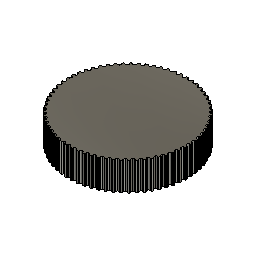
gear_67z (Autodesk Fusion 360 design; units mm, degrees)
Autodesk Fusion 360 part; units mm, degrees
sketch "Sketch1" plane through (0, 0, 0) normal (0, 0, 1) x (1, 0, 0) in component "gt2 pulley"
  circle A0 centre (0, 0) radius 21.3268 construction
  circle A1 centre (0, 0) radius 20.3228 construction
  line L0 (0, 0) -> (0, 21.3268) construction
  line L1 (0, 0) -> (0.9996, 21.3033) construction
  line L2 (0, 0) -> (1.4057, 21.2804) construction
  circle A2 centre (0, 0) radius 21.0728 construction
  arc A3 (0.3932, 20.9351) -> (0.4668, 20.6401) centre (1.389, 21.0269) ccw
  circle A4 centre (0, 0) radius 20.9228 construction
  arc A5 (0.2455, 21.0713) -> (0, 21.0728) centre (0, 0) ccw
  arc A6 (0.3932, 20.9351) -> (0.2455, 21.0713) centre (0.2438, 20.9213) ccw
  arc A7 (0.4668, 20.6401) -> (0.9526, 20.3004) centre (0.9786, 20.8548) ccw
  arc A8 (0, 21.0728) -> (-0.2455, 21.0713) centre (0, 0) ccw
  arc A9 (-0.2455, 21.0713) -> (-0.3932, 20.9351) centre (-0.2438, 20.9213) ccw
  arc A10 (-0.4668, 20.6401) -> (-0.3932, 20.9351) centre (-1.389, 21.0269) ccw
  arc A11 (-0.9524, 20.3004) -> (-0.4668, 20.6401) centre (-0.9786, 20.8548) ccw
  arc A12 (0.9526, 20.3004) -> (-0.9526, 20.3004) centre (0, 0) ccw
  point P0 (1.389, 21.0269)
  point P1 (0, 21.0728)
  dimension "d18" = 42.6535
  dimension "d19" = 2.687
  dimension "d22" = 1.004
  dimension "d24" = 0.75
  dimension "d26" = 1
  dimension "d27" = 0.15
  dimension "d28" = 0.15
  dimension "d47" = 0.555
  dimension "d52" = 3.812
  constraint coincident A0.centre A1.centre
  constraint coincident A0 L0.end
  constraint vertical L0
  constraint coincident A0 L1.end
  constraint coincident A0 L2.end
  constraint concentric A1 A2
  constraint coincident A1 A7.end
  constraint coincident L1 A7.end
  constraint coincident A2 P0
  constraint coincident L2 P0
  constraint coincident P0 A3.centre
  constraint coincident A2 P1
  constraint coincident L0 P1
  constraint concentric A2 A4
  constraint coincident P1 A5.end
  constraint coincident A4 A6.centre
  constraint coincident A3.start A6.start
  constraint tangent A3 A6
  constraint tangent A3 A7
  constraint symmetric L0 A7.end A12.end
  constraint symmetric L0 A3.start A9.end
  constraint symmetric L0 A3.end A10.start
  constraint symmetric L0 A3 A10
  constraint symmetric L0 A5.start A8.end
  constraint symmetric L0 P1 A5.end
  constraint symmetric L0 A5 A8
  constraint symmetric L0 A6 A9
  constraint symmetric L0 A7 A11
  constraint coincident A1 A11.start
  constraint tangent A1 A7
  constraint coincident L1 A7.centre
  measures "d18" diameter of A0
  measures "d19" angle of L0 L1
  measures "d22" distance of A0 A1
  measures "d24" distance of A1 A2
  measures "d26" radius of A3
  measures "d27" distance of A2 A4
  measures "d28" radius of A6
  measures "d47" radius of A7
extrude "Extrude1" add sketch "Sketch1" along normal blind 10 makes body 1
pattern_circular "C-Pattern1" count 67 over 360 about axis through (0, 0, 1.75) along (0, 0, 1) of bodies 1 makes body 2 at (-2.6393, 20.1506, 6.6667) makes body 3 at (-4.5147, 19.815, 6.6667) makes body 4 at (-6.3503, 19.3051, 6.6667) makes body 5 at (-7.5442, 18.8706, 6.6667) makes body 6 at (-9.2781, 18.0813, 6.6667) makes body 7 at (-10.2072, 17.5735, 3.3333) makes body 8 at (-12.9818, 15.6361, 6.6667) makes body 9 at (-14.3889, 14.3518, 6.6667) makes body 10 at (-15.2575, 13.4247, 6.6667) makes body 11 at (-16.8126, 11.4171, 6.6667) makes body 12 at (-17.4931, 10.3443, 6.6667) makes body 13 at (-18.0081, 9.4192, 3.3333) makes body 14 at (-19.3215, 6.3004, 6.6667) makes body 15 at (-19.8266, 4.4634, 6.6667) makes body 16 at (-20.0667, 3.2159, 6.6667) makes body 17 at (-20.3111, 0.6883, 6.6667) makes body 18 at (-20.2863, -1.2167, 6.6667) makes body 19 at (-20.0832, -3.111, 6.6667) makes body 20 at (-19.8496, -4.3598, 6.6667) makes body 21 at (-19.3541, -6.1994, 6.6667) makes body 22 at (-19.005, -7.1989, 3.3333) makes body 23 at (-17.8588, -9.6994, 6.6667) makes body 24 at (-16.6323, -11.6782, 6.6667) makes body 25 at (-15.3275, -13.3448, 6.6667) makes body 26 at (-14.4637, -14.2764, 6.6667) makes body 27 at (-12.5704, -15.9687, 6.6667) makes body 28 at (-12.2348, -16.2273, 3.3333) makes body 29 at (-9.3724, -18.0325, 6.6667) makes body 30 at (-8.9945, -18.224, 3.3333) makes body 31 at (-6.0482, -19.4019, 6.6667) makes body 32 at (-4.6182, -19.7911, 6.6667) makes body 33 at (-2.114, -20.2125, 6.6667) makes body 34 at (-0.2119, -20.3217, 6.6667) makes body 35 at (1.6919, -20.2522, 6.6667) makes body 36 at (3.581, -20.0048, 6.6667) makes body 37 at (5.4385, -19.5816, 6.6667) makes body 38 at (7.2482, -18.9862, 6.6667) makes body 39 at (7.6425, -18.831, 3.3333) makes body 40 at (9.3722, -18.0326, 3.3333) makes body 41 at (11.7215, -16.6018, 6.6667) makes body 42 at (13.7004, -15.0104, 6.6667) makes body 43 at (15.0458, -13.6615, 6.6667) makes body 44 at (16.259, -12.1926, 6.6667) makes body 45 at (17.3293, -10.6165, 6.6667) makes body 46 at (17.9588, -9.513, 6.6667) makes body 47 at (18.4298, -8.5648, 3.3333) makes body 48 at (19.3541, -6.1996, 6.6667) makes body 49 at (20.014, -3.5292, 6.6667) makes body 50 at (20.2565, -1.6395, 6.6667) makes body 51 at (20.321, 0.2645, 6.6667) makes body 52 at (20.207, 2.1662, 6.6667) makes body 53 at (20.0321, 3.4246, 6.6667) makes body 54 at (19.4487, 5.896, 6.6667) makes body 55 at (19.0423, 7.0997, 6.6667) makes body 56 at (18.2938, 8.8517, 6.6667) makes body 57 at (17.0471, 11.064, 6.6667) makes body 58 at (16.8127, 11.4169, 3.3333) makes body 59 at (14.8307, 13.8948, 3.3333) makes body 60 at (13.3051, 15.3619, 6.6667) makes body 61 at (11.8081, 16.5404, 6.6667) makes body 62 at (10.2074, 17.5734, 6.6667) makes body 63 at (9.0894, 18.1768, 6.6667) makes body 64 at (7.3473, 18.9481, 6.6667) makes body 65 at (5.7441, 19.4941, 6.6667) makes body 66 at (3.059, 20.0912, 6.6667) makes body 67 at (2.6396, 20.1506, 3.3333)
sketch "Sketch2" plane through (0, 0, 10) normal (0, 0, 1) x (-1, 0, 0)
  arc A0 (-14.5613, -15.0466) -> (-14.5462, -15.247) centre (-14.4427, -15.1384) ccw
  arc A1 (-14.5462, -15.247) -> (-14.187, -15.5817) centre (0, 0) ccw
  arc A2 (-14.187, -15.5817) -> (-13.9861, -15.5828) centre (-14.086, -15.4708) ccw
  arc A3 (-13.7311, -15.4172) -> (-13.9861, -15.5828) centre (-13.3203, -16.3289) ccw
  arc A4 (-13.1443, -15.4997) -> (-13.7311, -15.4172) centre (-13.5031, -15.9232) ccw
  arc A5 (-14.5378, -14.2009) -> (-13.1443, -15.4997) centre (0, 0) ccw
  arc A6 (-14.4141, -14.7807) -> (-14.5378, -14.2009) centre (-14.9348, -14.5887) ccw
  arc A7 (-14.5613, -15.0466) -> (-14.4141, -14.7807) centre (-15.3524, -14.4349) ccw
  circle A8 centre (0, 0) radius 20.3228
  constraint coincident A1.centre A5.centre
extrude "Extrude2" add sketch "Sketch2" against normal blind 10 contours A5 A8 bodies 1 2 3 4 5 6 7 8 9 10 11 12 13 14 15 16 17 18 19 20 21 22 23 24 25 26 27 28 29 30 31 32 33 34 35 36 37 38 39 40 41 42 43 44 45 46 47 48 49 50 51 52 53 54 55 56 57 58 59 60 61 62 63 64 65 66 67
extrude "Extrude4" [suppressed] in component "gt2 pulley"
pattern_circular "C-Pattern7" [suppressed] in component "gt2 pulley"
extrude "Extrude3" [suppressed] in component "gt2 pulley"
pattern_circular "C-Pattern6" [suppressed] in component "gt2 pulley"
extrude "Extrude2'" [suppressed] in component "gt2 pulley"
pattern_circular "C-Pattern5" [suppressed] in component "gt2 pulley"
extrude "Extrude1'" [suppressed] in component "gt2 pulley"
pattern_circular "C-Pattern4" [suppressed] in component "gt2 pulley"
pattern_circular "C-Pattern3" [suppressed] in component "gt2 pulley"
pattern_circular "C-Pattern2" [suppressed] in component "gt2 pulley"
pattern_circular "C-Pattern1'" [suppressed] in component "gt2 pulley"
copy_body "Body->Comp1" [suppressed] in component "Component"
copy_body "Body->Comp2" [suppressed] in component "Component'"
copy_body "Body->Comp3" [suppressed] in component "Component''"
copy_body "Body->Comp4" [suppressed] in component "Component'''"
copy_body "Body->Comp5" [suppressed] in component "Component''''"
copy_body "Body->Comp6" [suppressed] in component "Component'''''"
copy_body "Body->Comp7" [suppressed] in component "Component''''''"
copy_body "Body->Comp8" [suppressed] in component "Component'''''''"
copy_body "Body->Comp9" [suppressed] in component "Component''''''''"
copy_body "Body->Comp10" [suppressed] in component "Component'''''''''"
copy_body "Body->Comp11" [suppressed] in component "Component''''''''''"
copy_body "Body->Comp12" [suppressed] in component "Component'''''''''''"
copy_body "Body->Comp13" [suppressed] in component "Component''''''''''''"
copy_body "Body->Comp14" [suppressed] in component "Component'''''''''''''"
copy_body "Body->Comp15" [suppressed] in component "Component''''''''''''''"
copy_body "Body->Comp16" [suppressed] in component "Component'''''''''''''''"
copy_body "Body->Comp17" [suppressed] in component "Component''''''''''''''''"
copy_body "Body->Comp18" [suppressed] in component "Component'''''''''''''''''"
copy_body "Body->Comp19" [suppressed] in component "Component''''''''''''''''''"
copy_body "Body->Comp20" [suppressed] in component "Component'''''''''''''''''''"
component "gt2 pulley" placed x (1, 0, 0) y (0, 1, 0) z (0, 0, 1) at (0, 0, 0)
equation "NumTeeth = 67" comment "min 20"
equation "ToothPitch = 2 mm"
equation "PullyDia = NumTeeth * ToothPitch / PI"
equation "ToothAng = ( ( 360 / NumTeeth ) * 1 deg )"
equation "TransOffsetAngle = ToothAng * 0.2"
equation "Sholulder_Radius = 0.15 mm"
equation "Root_Radius = 0.555 mm"
equation "TransRadius = 1 mm"
equation "ToolHeight = 0.75 mm"
equation "PLD = 0.254 mm"
equation "d18 = PullyDia"
equation "d19 = ToothAng / 2"
equation "d22 = PLD + ToolHeight"
equation "d24 = ToolHeight"
equation "d26 = TransRadius"
equation "d27 = Sholulder_Radius"
equation "d31 = NumTeeth"
equation "d33 = NumTeeth"
equation "d35 = NumTeeth"
equation "d37 = NumTeeth"
equation "d41 = NumTeeth"
equation "d45 = NumTeeth"
equation "d47 = Root_Radius"
equation "d50 = NumTeeth"
